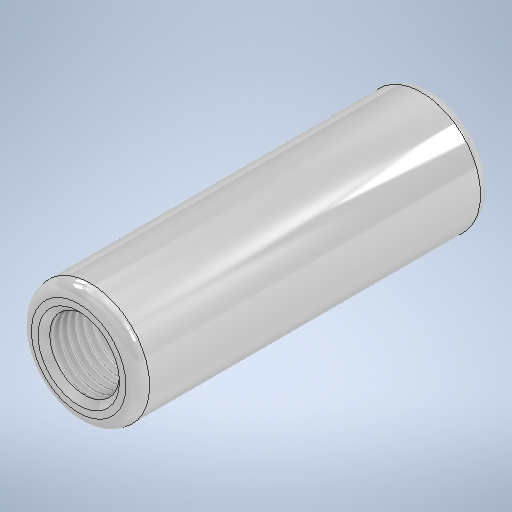
# Autodesk Inventor part: Plenum
Saved by Autodesk Inventor 2025.2 (Build 292293000, 293)
## iProperties
Created: 2026-06-25
Part Number: Plenum
Material: Generic
Document SubType Name: Modeling
Designer: Simon
Density: 1 g/cm^3
Appearance: Aluminum - Polished
Author: Simon
Autodesk Inventor part; units mm, degrees
ref_plane "YZ Plane" through (0, 0, 0) normal (1, 0, 0) x (0, 1, 0)
ref_plane "XZ Plane" through (0, 0, 0) normal (0, 1, 0) x (-1, 0, 0)
ref_plane "XY Plane" through (0, 0, 0) normal (0, 0, 1) x (1, 0, 0)
sketch "Sketch1" plane through (0, 0, 0) normal (0, 0, 1) x (1, 0, 0)
  circle A0 centre (0, 0) radius 5.9
  circle A1 centre (0, 0) radius 10
  dimension "d0" = 11.8
  dimension "d1" = 20
  constraints: 2 centre point, 2 coincident
  measures "d0" diameter of A0
  measures "d1" diameter of A1
extrude "Extrusion1" add sketch "Sketch1" along normal mid plane 60
thread "Thread1" size "G 1/4-19" standard "BSP Pipe Threads" length 10
thread "Thread2" size "G 1/4-19" standard "BSP Pipe Threads" length 10
chamfer "Chamfer1" distance 1 angle 45 2 edges at (-5.9, 0, 30) (-5.9, 0, -30)
fillet "Fillet1" radius 2 2 edges at (-10, 0, -30) (-10, 0, 30)
body "Solid1"
